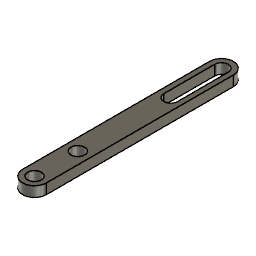
BRAZO_DIRECCION (Autodesk Fusion 360 design; units mm, degrees)
Autodesk Fusion 360 part; units mm, degrees
sketch "Boceto1" plane through (0, 0, 0) normal (0, 0, 1) x (1, 0, 0)
  line L0 (-25.6714, 0) -> (25.6714, 0) construction
  line L1 (0, -23) -> (0, 29) construction
  line L2 (-3.5, 21.001) -> (3.5, 21.001) construction
  line L3 (-4, 25.5) -> (4, 25.5) construction
  arc A0 (3.5, 25.5) -> (-3.5, 25.5) centre (0, 25.5) ccw
  line L4 (-3.5, 25.5) -> (-3.5, -29.5)
  line L5 (3.5, 25.5) -> (3.5, -29.5)
  line L6 (-4, -29.5) -> (4, -29.5) construction
  arc A1 (-3.5, -29.5) -> (3.5, -29.5) centre (0, -29.5) ccw
  circle A2 centre (0, -29.5) radius 2
  circle A3 centre (0, -16.762) radius 2
  line L7 (-1.9722, 25.5) -> (-1.9722, 10.5)
  line L8 (2.0278, 25.5) -> (2.0278, 10.5)
  arc A4 (2.0278, 25.5) -> (-1.9722, 25.5) centre (0.0278, 25.5) ccw
  arc A5 (-1.9722, 10.5) -> (2.0278, 10.5) centre (0.0278, 10.5) ccw
  point P0 (-3.5, 0)
  point P1 (3.5, -0.1376)
  point P2 (0, 21.001)
  point P3 (0, 21.001)
  point P4 (0, -33)
  dimension "d4" = 7
  dimension "d6" = 4
  dimension "d7" = 4
  dimension "d8" = 12.738
  dimension "d9" = 15
  dimension "d10" = 15
  dimension "d11" = 4
  dimension "d14" = 55
  dimension "d15" = 62
  constraint vertical L4
  constraint midpoint L0 origin
  constraint perpendicular L0 L4
  constraint perpendicular L0 L1
  constraint parallel L1 L5
  constraint coincident L2.start L4
  constraint perpendicular L2 L4
  constraint coincident L2.end L5
  constraint midpoint L2 P3
  constraint coincident P3 P2
  constraint coincident L1 P3
  constraint coincident P0 L4
  constraint coincident L1 origin
  constraint coincident P1 L5
  constraint perpendicular L3 L5
  constraint coincident L3 A0.end
  constraint coincident L3 A0.start
  constraint tangent A0 L4
  constraint midpoint L1.end A0
  constraint perpendicular L5 L6
  constraint coincident L6 L4.end
  constraint coincident L6 L5.end
  constraint tangent L4 A1
  constraint concentric A1 A2
  constraint coincident L1 A3.centre
  constraint parallel L4 L7
  constraint perpendicular L2 L8
  constraint coincident L3 L7.start
  constraint coincident L3 L8.start
  constraint tangent L7 A4
  constraint tangent L7 A5
  constraint midpoint A1 P4
  measures "d4" distance of L4 L5
  measures "d6" diameter of A2
  measures "d7" diameter of A3
  measures "d8" distance of A1.centre A3.centre
  measures "d9" distance of L7.start L7.end
  measures "d10" distance of L8.start L8.end
  measures "d11" distance of L7 L8
  measures "d14" distance of A0.start L5.end
  measures "d15" distance of L1.end P4
extrude "Extruir1" add sketch "Boceto1" along normal blind 3
